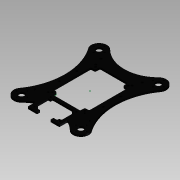
# Autodesk Inventor part: baseatasV2
Saved by Autodesk Inventor 2015 SP1 (Build 190203100, 203)
## iProperties
Created: 2015-01-15
Part Number: baseatasV2
Material: ABS Plastic
Document SubType Name: Modeling
Designer: Rafi Kurnia Putra
Density: 1.06 g/cm^3
Appearance: Smooth - Black
Mass: 28.287 g
Surface Area: 202.895 cm^2
Volume: 26.6858 cm^3
Author: Rafi Kurnia Putra
Autodesk Inventor part; units mm, degrees
ref_plane "YZ Plane" through (0, 0, 0) normal (1, 0, 0) x (0, 1, 0)
ref_plane "XZ Plane" through (0, 0, 0) normal (0, 1, 0) x (-1, 0, 0)
ref_plane "XY Plane" through (0, 0, 0) normal (0, 0, 1) x (1, 0, 0)
sketch "Sketch1" plane through (0, 0, 0) normal (0, 1, 0) x (-1, 0, 0)
  circle A0 centre (-25.375, -42.175) radius 1.75
  circle A1 centre (-25.375, -42.175) radius 1.75
  circle A2 centre (-28.625, -37.55) radius 1.75
  circle A3 centre (-28.625, -37.55) radius 1.75
  circle A4 centre (-25.5, -34.24) radius 1.75
  circle A5 centre (-46.65, -60.8866) radius 4.5
  circle A6 centre (-46.65, -69.3733) radius 1.25
  circle A7 centre (-38.1633, -60.8866) radius 1.25
  circle A8 centre (-55.1367, -60.8866) radius 1.25
  circle A9 centre (-46.65, -52.3999) radius 1.25
  circle A10 centre (-39.5789, -53.8156) radius 1.25
  circle A11 centre (-33.215, -47.4516) radius 1.25
  line L0 (0, -37.55) -> (-19.7877, -37.55)
  line L1 (-21.7877, -35.55) -> (-21.7877, -32)
  line L2 (-28.625, -28) -> (-28.625, 0)
  arc A12 (-28.625, -28) -> (-26.625, -30) centre (-26.625, -28) ccw
  line L3 (-23.7877, -30) -> (-26.625, -30)
  arc A13 (-21.7877, -32) -> (-23.7877, -30) centre (-23.7877, -32) ccw
  arc A14 (-21.7877, -35.55) -> (-19.7877, -37.55) centre (-19.7877, -35.55) ccw
  arc A15 (-21.37, 36.7732) -> (-21.7877, 35.55) centre (-19.7877, 35.55) ccw
  circle A16 centre (-28.625, 37.55) radius 1.75
  circle A17 centre (-28.625, 37.55) radius 1.75
  circle A18 centre (-33.215, 47.4516) radius 1.25
  circle A19 centre (-38.1633, 60.8866) radius 1.25
  circle A20 centre (-39.5789, 53.8156) radius 1.25
  circle A21 centre (-46.65, 52.3999) radius 1.25
  circle A22 centre (-46.65, 69.3733) radius 1.25
  circle A23 centre (-46.65, 60.8866) radius 4.5
  circle A24 centre (-55.1367, 60.8866) radius 1.25
  circle A25 centre (-25.5, 34.24) radius 1.75
  line L4 (-21.7877, 35.55) -> (-21.7877, 32)
  line L5 (-23.7877, 30) -> (-26.625, 30)
  arc A26 (-26.625, 30) -> (-28.625, 28) centre (-26.625, 28) ccw
  line L6 (-28.625, 28) -> (-28.625, 0)
  arc A27 (-23.7877, 30) -> (-21.7877, 32) centre (-23.7877, 32) ccw
  circle A28 centre (-34.6272, 13.8987) radius 1.75
  circle A29 centre (-35.7091, 28.8987) radius 1.75
  circle A30 centre (-25.5, 34.24) radius 1.75
  circle A31 centre (-28.625, 37.55) radius 1.75
  circle A32 centre (-38.6257, 37.55) radius 1.75
  arc A33 (-37.9702, 69.5664) -> (-55.3297, 52.2069) centre (-46.65, 60.8866) ccw
  circle A34 centre (-34.6272, -13.8987) radius 1.75
  circle A35 centre (-25.5, -34.24) radius 1.75
  circle A36 centre (-28.625, -37.55) radius 1.75
  circle A37 centre (-25.375, -42.175) radius 1.75
  arc A38 (-55.3297, -52.2069) -> (-37.9702, -69.5664) centre (-46.65, -60.8866) ccw
  circle A39 centre (-28.8757, 53.55) radius 1.75
  arc A40 (-37.9702, 69.5664) -> (-26.4933, 60.8302) centre (-0.0022, 107.5388) ccw
  arc A41 (0, -40.4412) -> (0, -43.9412) centre (0, -42.1912) ccw
  arc A42 (0, -53.835) -> (-37.9702, -69.5664) centre (0, -107.5245) ccw
  arc A43 (-55.3297, -52.2069) -> (-55.3297, 52.2069) centre (-134.1138, 0) ccw
  arc A44 (0, -46.2631) -> (0, -49.7631) centre (0, -48.0131) ccw
  line L7 (-39.6019, 0) -> (-25.7032, 0) construction
  arc A45 (23.7877, -30) -> (21.7877, -32) centre (23.7877, -32) ccw
  line L8 (28.625, -28) -> (28.625, 0)
  line L9 (21.7877, -35.55) -> (21.7877, -32)
  arc A46 (19.7877, -37.55) -> (21.7877, -35.55) centre (19.7877, -35.55) ccw
  arc A47 (26.625, -30) -> (28.625, -28) centre (26.625, -28) ccw
  circle A48 centre (25.5, -34.24) radius 1.75
  circle A49 centre (28.625, -37.55) radius 1.75
  circle A50 centre (28.625, -37.55) radius 1.75
  circle A51 centre (25.375, -42.175) radius 1.75
  circle A52 centre (25.375, -42.175) radius 1.75
  line L10 (0, -37.55) -> (19.7877, -37.55)
  circle A53 centre (46.65, -60.8866) radius 4.5
  circle A54 centre (46.65, -69.3733) radius 1.25
  circle A55 centre (38.1633, -60.8866) radius 1.25
  circle A56 centre (55.1367, -60.8866) radius 1.25
  circle A57 centre (46.65, -52.3999) radius 1.25
  circle A58 centre (33.215, -47.4516) radius 1.25
  circle A59 centre (39.5789, -53.8156) radius 1.25
  line L11 (23.7877, -30) -> (26.625, -30)
  circle A60 centre (38.1633, 60.8866) radius 1.25
  circle A61 centre (39.5789, 53.8156) radius 1.25
  circle A62 centre (46.65, 52.3999) radius 1.25
  circle A63 centre (55.1367, 60.8866) radius 1.25
  circle A64 centre (46.65, 60.8866) radius 4.5
  circle A65 centre (46.65, 69.3733) radius 1.25
  line L12 (28.625, 28) -> (28.625, 0)
  line L13 (23.7877, 30) -> (26.625, 30)
  arc A66 (28.625, 28) -> (26.625, 30) centre (26.625, 28) ccw
  arc A67 (21.7877, 32) -> (23.7877, 30) centre (23.7877, 32) ccw
  line L14 (21.7877, 35.55) -> (21.7877, 32)
  arc A68 (21.7877, 35.55) -> (21.37, 36.7732) centre (19.7877, 35.55) ccw
  circle A69 centre (25.5, 34.24) radius 1.75
  circle A70 centre (28.625, 37.55) radius 1.75
  circle A71 centre (28.625, 37.55) radius 1.75
  circle A72 centre (33.215, 47.4516) radius 1.25
  arc A73 (55.3297, 52.2069) -> (37.9702, 69.5664) centre (46.65, 60.8866) ccw
  circle A74 centre (25.5, 34.24) radius 1.75
  circle A75 centre (34.6272, 13.8987) radius 1.75
  circle A76 centre (35.7091, 28.8987) radius 1.75
  arc A77 (55.3297, 52.2069) -> (55.3297, -52.2069) centre (134.1138, 0) ccw
  circle A78 centre (34.6272, -13.8987) radius 1.75
  circle A79 centre (28.625, 37.55) radius 1.75
  circle A80 centre (38.6257, 37.55) radius 1.75
  circle A81 centre (25.5, -34.24) radius 1.75
  circle A82 centre (28.625, -37.55) radius 1.75
  circle A83 centre (25.375, -42.175) radius 1.75
  arc A84 (0, -43.9412) -> (0, -40.4412) centre (0, -42.1912) ccw
  arc A85 (37.9702, -69.5664) -> (0, -53.835) centre (0, -107.5245) ccw
  arc A86 (37.9702, -69.5664) -> (55.3297, -52.2069) centre (46.65, -60.8866) ccw
  circle A87 centre (28.8757, 53.55) radius 1.75
  arc A88 (26.4933, 60.8302) -> (37.9702, 69.5664) centre (0.0022, 107.5388) ccw
  arc A89 (0, -49.7631) -> (0, -46.2631) centre (0, -48.0131) ccw
  line L15 (39.6019, 0) -> (25.7032, 0) construction
  line L16 (0, 0) -> (146.4608, 0) construction
  line L17 (-25, 72.1616) -> (-25, 61.7)
  line L18 (-20.5788, 37.1616) -> (20.5788, 37.1616)
  line L19 (25, 61.7) -> (25, 72.1616)
  circle A90 centre (20, 68.1616) radius 1.75
  circle A91 centre (-20, 68.1616) radius 1.75
  circle A92 centre (20, 42.1616) radius 1.75
  circle A93 centre (-20, 42.1616) radius 1.75
  line L20 (10, 72.1616) -> (10, 69.1616)
  line L21 (-10.74, 69.1616) -> (-10.74, 72.1616)
  arc A94 (-26.4933, 60.8302) -> (-25, 61.7) centre (-26, 61.7) ccw
  arc A95 (25, 61.7) -> (26.4933, 60.8302) centre (26, 61.7) ccw
  line L22 (24, 73.1616) -> (11, 73.1616)
  line L23 (-24, 73.1616) -> (-11.74, 73.1616)
  arc A96 (21.37, 36.7732) -> (20.5788, 37.1616) centre (20.5788, 36.1616) ccw
  arc A97 (-20.5788, 37.1616) -> (-21.37, 36.7732) centre (-20.5788, 36.1616) ccw
  line L24 (20, 63.6616) -> (20, 46.6616)
  line L25 (-16.5, 67.1616) -> (-16.5, 65.6616)
  line L26 (-17.5, 64.6616) -> (-19, 64.6616)
  line L27 (-20, 63.6616) -> (-20, 46.6616)
  line L28 (-19, 45.6616) -> (-17.5, 45.6616)
  line L29 (-16.5, 44.6616) -> (-16.5, 43.1616)
  line L30 (-15.5, 42.1616) -> (15.5, 42.1616)
  line L31 (16.5, 43.1616) -> (16.5, 44.6616)
  line L32 (17.5, 45.6616) -> (19, 45.6616)
  line L33 (16.5, 67.1616) -> (16.5, 65.6616)
  line L34 (17.5, 64.6616) -> (19, 64.6616)
  line L35 (15.5, 68.1616) -> (11, 68.1616)
  line L36 (-11.74, 68.1616) -> (-15.5, 68.1616)
  arc A98 (19, 45.6616) -> (20, 46.6616) centre (19, 46.6616) ccw
  arc A99 (17.5, 45.6616) -> (16.5, 44.6616) centre (17.5, 44.6616) ccw
  arc A100 (15.5, 42.1616) -> (16.5, 43.1616) centre (15.5, 43.1616) ccw
  arc A101 (-16.5, 43.1616) -> (-15.5, 42.1616) centre (-15.5, 43.1616) ccw
  arc A102 (-16.5, 44.6616) -> (-17.5, 45.6616) centre (-17.5, 44.6616) ccw
  arc A103 (-20, 46.6616) -> (-19, 45.6616) centre (-19, 46.6616) ccw
  arc A104 (20, 63.6616) -> (19, 64.6616) centre (19, 63.6616) ccw
  arc A105 (16.5, 67.1616) -> (15.5, 68.1616) centre (15.5, 67.1616) ccw
  arc A106 (16.5, 65.6616) -> (17.5, 64.6616) centre (17.5, 65.6616) ccw
  arc A107 (10, 69.1616) -> (11, 68.1616) centre (11, 69.1616) ccw
  arc A108 (11, 73.1616) -> (10, 72.1616) centre (11, 72.1616) ccw
  arc A109 (25, 72.1616) -> (24, 73.1616) centre (24, 72.1616) ccw
  arc A110 (-10.74, 72.1616) -> (-11.74, 73.1616) centre (-11.74, 72.1616) ccw
  arc A111 (-11.74, 68.1616) -> (-10.74, 69.1616) centre (-11.74, 69.1616) ccw
  arc A112 (-15.5, 68.1616) -> (-16.5, 67.1616) centre (-15.5, 67.1616) ccw
  arc A113 (-17.5, 64.6616) -> (-16.5, 65.6616) centre (-17.5, 65.6616) ccw
  arc A114 (-19, 64.6616) -> (-20, 63.6616) centre (-19, 63.6616) ccw
  arc A115 (-24, 73.1616) -> (-25, 72.1616) centre (-24, 72.1616) ccw
  point P0 (-37.9702, -69.5664)
  point P1 (-55.3297, -52.2069)
  point P2 (-4.2075, -54.5249)
  point P3 (-46.65, -60.8866)
  point P4 (-37.9702, 69.5664)
  point P5 (-55.3297, 52.2069)
  point P6 (0.0035, -53.835)
  point P7 (-57.609, 54.4281)
  point P8 (-40.6295, 13.8987)
  point P9 (-40.6295, -13.8987)
  point P10 (55.3297, -52.2069)
  point P11 (37.9702, -69.5664)
  point P12 (37.9702, 69.5664)
  point P13 (55.3297, 52.2069)
  point P14 (46.65, -60.8866)
  point P15 (4.2075, -54.5249)
  point P16 (-0.0035, -53.835)
  point P17 (57.609, 54.4281)
  point P18 (40.6295, 13.8987)
  point P19 (40.6295, -13.8987)
  point P20 (-1.75, -48.0131)
  point P21 (25, 73.1616)
  point P22 (-25, 73.1616)
  point P23 (20.972, 37.1616)
  point P24 (-20.972, 37.1616)
  point P25 (25, 60.0142)
  point P26 (-25, 60.0142)
  point P27 (10, 68.1616)
  point P28 (-10, 68.1616)
  point P29 (10, 73.1616)
  point P30 (-10.74, 73.1616)
  point P31 (10, 68.1616)
  point P32 (20, 45.6616)
  point P33 (20, 64.6616)
  point P34 (16.5, 42.1616)
  point P35 (-16.5, 42.1616)
  point P36 (-16.5, 68.1616)
  point P37 (16.5, 68.1616)
  point P38 (-16.5, 45.6616)
  point P39 (16.5, 45.6616)
  point P40 (46.65, -73.1616)
  point P41 (-58.925, -60.8866)
  point P42 (58.925, -60.8866)
  dimension "d42" = 9
  dimension "d43" = 9
  dimension "d46" = 2.5
  dimension "d86" = 12.0045
  dimension "d87" = 6.0022
  dimension "d88" = 6.0022
  dimension "d92" = 69.2545
  dimension "d93" = 27.7974
  dimension "d94" = 5.8219
  dimension "d95" = 5.8219
  dimension "d97" = 68.48
  dimension "d98" = 51
  dimension "d99" = 9
  dimension "d100" = 8.4867
  dimension "d101" = 2.5
  dimension "d102" = 10
  dimension "d103" = 9
  dimension "d104" = 8.4867
  dimension "d112" = 90
  dimension "d113" = 3.5
  dimension "d114" = 5
  dimension "d116" = 3.5
  dimension "d117" = 5
  dimension "d119" = 3.5
  dimension "d120" = 5
  dimension "d121" = 5
  dimension "d122" = 3.5
  dimension "d123" = 5
  dimension "d124" = 5
  dimension "d126" = 10
  dimension "d133" = 1
  dimension "d137" = 1
  dimension "d138" = 3.5
  dimension "d139" = 3.5
  dimension "d140" = 3.5
  dimension "d141" = 3.5
  dimension "d142" = 1
  dimension "d143" = 3.5
  dimension "d144" = 3.5
  dimension "d145" = 3.5
  dimension "d146" = 1
  dimension "d170" = 146.3233
  dimension "d171" = 117.85
  constraints: 116 centre point, 112 point on circle, 74 end point, 44 tangent, 32 point on line, 18 equal radius, 12 coincident, 11 perpendicular, 6 horizontal, 4 vertical, 4 other
  measures "d42" diameter of A5
  measures "d43" diameter of A23
  measures "d46" diameter of A8
  measures "d86" distance from line of L6 point (-40.629, 13.899)
  measures "d87" distance of A28.centre point (-40.629, 13.899)
  measures "d88" distance of A34.centre point (-40.629, -13.899)
  measures "d92" distance of A28.centre A75.centre
  measures "d93" distance of A78.centre A75.centre
  measures "d94" distance of A44.centre point (0.004, -53.835)
  measures "d95" distance of A84.centre A44.centre
  measures "d97" distance of A81.centre A74.centre
  measures "d98" distance of A25.centre A74.centre
  measures "d99" diameter of A64
  measures "d100" distance of A63.centre A64.centre
  measures "d101" diameter of A63
  measures "d102" distance of A61.centre A64.centre
  measures "d103" distance of A72.centre A61.centre
  measures "d104" distance of A60.centre A73.centre
  measures "d112" angle of L18 L17
  measures "d113" diameter of A90
  measures "d114" distance from line of A90.centre L19
  measures "d116" diameter of A91
  measures "d117" distance from line of L17 A91.centre
  measures "d119" diameter of A92
  measures "d120" distance from line of A92.centre L19
  measures "d121" distance from line of A92.centre L18
  measures "d122" diameter of A93
  measures "d123" distance from line of A93.centre L18
  measures "d124" distance from line of A93.centre L17
  measures "d126" distance of point (-10, 68.162) A91.centre
  measures "d133" radius of A94
  measures "d137" radius of A96
  measures "d138" distance of point (20, 45.662) A92.centre
  measures "d139" distance of point (20, 64.662) A90.centre
  measures "d140" distance of point (16.5, 42.162) A92.centre
  measures "d141" distance of point (-16.5, 42.162) A93.centre
  measures "d142" radius of A98
  measures "d143" distance from line of A91.centre L26
  measures "d144" distance of point (16.5, 68.162) A90.centre
  measures "d145" distance of A91.centre point (-16.5, 68.162)
  measures "d146" radius of A104
  measures "d170" distance from line of point (46.65, -73.162) L22
  measures "d171" distance of point (-58.925, -60.887) point (58.925, -60.887)
extrude "Extrusion6" add sketch "Sketch1" along normal mid plane 3
sketch "Sketch5" plane through (0, 1.5, 0) normal (0, 1, 0) x (1, 0, 0)
  line L0 (-68.183, -17.0535) -> (-47.8943, -30.2678)
  arc A0 (-46.3635, -35.1053) -> (-46.3635, 35.1053) centre (-134.1138, 0) ccw
  line L1 (-68.183, 17.0535) -> (-47.8943, 30.2678)
  arc A1 (-46.3635, -35.1053) -> (-47.8943, -30.2678) centre (-50.0774, -33.6196) ccw
  arc A2 (-47.8943, 30.2678) -> (-46.3635, 35.1053) centre (-50.0774, 33.6196) ccw
  line L2 (0, -8.7241) -> (0, 8.1787)
  line L3 (-70, -13.7017) -> (-70, 13.7017)
  arc A3 (-68.183, 17.0535) -> (-70, 13.7017) centre (-66, 13.7017) ccw
  arc A4 (-70, -13.7017) -> (-68.183, -17.0535) centre (-66, -13.7017) ccw
  line L4 (68.183, -17.0535) -> (47.8943, -30.2678)
  arc A5 (46.3635, 35.1053) -> (46.3635, -35.1053) centre (134.1138, 0) ccw
  line L5 (68.183, 17.0535) -> (47.8943, 30.2678)
  arc A6 (47.8943, -30.2678) -> (46.3635, -35.1053) centre (50.0774, -33.6196) ccw
  arc A7 (46.3635, 35.1053) -> (47.8943, 30.2678) centre (50.0774, 33.6196) ccw
  line L6 (70, -13.7017) -> (70, 13.7017)
  arc A8 (70, 13.7017) -> (68.183, 17.0535) centre (66, 13.7017) ccw
  arc A9 (68.183, -17.0535) -> (70, -13.7017) centre (66, -13.7017) ccw
  point P0 (0, 0)
  point P1 (-45.1937, -32.0268)
  point P2 (-70, 0)
  point P3 (45.1937, -32.0268)
  point P4 (70, 0)
  dimension "d150" = 4
  dimension "d154" = 70
  dimension "d155" = 4
  constraints: 20 point on circle, 15 symmetric about line, 14 end point, 10 centre point, 6 tangent, 3 vertical, 2 equal radius, 2 point on line, 5 other
  measures "d150" radius of A1
  measures "d154" distance from line of point (-70, 0) L2
  measures "d155" radius of A3
sketch "Sketch7" plane through (0, 1.5, 0) normal (0, 1, 0) x (1, 0, 0)
  arc A0 (0, 53.835) -> (37.9702, 69.5664) centre (0, 107.5245) ccw
  arc A1 (-37.9702, 69.5664) -> (0, 53.835) centre (0, 107.5245) ccw
  arc A2 (46.65, 73.1616) -> (37.9702, 69.5664) centre (46.65, 60.8866) ccw
  arc A3 (-37.9702, 69.5664) -> (-46.65, 73.1616) centre (-46.65, 60.8866) ccw
  line L0 (46.65, 73.1616) -> (-46.65, 73.1616)
  constraints: 8 point on circle, 4 centre point, 2 end point, 1 horizontal
sketch "Sketch8" plane through (0, 1.5, 0) normal (0, 1, 0) x (1, 0, 0)
  arc A0 (55.3297, 52.2069) -> (55.3297, -52.2069) centre (134.1138, 0) ccw projected
  circle A1 centre (55.1367, -60.8866) radius 1.25 projected
  circle A2 centre (-55.1367, -60.8866) radius 1.25 projected
  arc A3 (-55.3297, -52.2069) -> (-37.9702, -69.5664) centre (-46.65, -60.8866) ccw projected
  circle A4 centre (46.65, 69.3733) radius 1.25 projected
  arc A5 (55.3297, 52.2069) -> (37.9702, 69.5664) centre (46.65, 60.8866) ccw projected
  line L0 (11.74, -73.1616) -> (24, -73.1616) projected
  circle A6 centre (35.7091, -28.8987) radius 1.75 projected
  circle A7 centre (-35.7091, -28.8987) radius 1.75 projected
  line L1 (0, 0) -> (-2.9258, 0)
  circle A8 centre (35.7091, 28.8987) radius 1.75
  circle A9 centre (-35.7091, 28.8987) radius 1.75
  circle A10 centre (38.6257, -37.55) radius 1.75 projected
  circle A11 centre (-38.6257, -37.55) radius 1.75 projected
  circle A12 centre (38.6257, 37.55) radius 1.75
  circle A13 centre (-38.6257, 37.55) radius 1.75
  point P0 (39.6019, 0)
  point P1 (-39.6104, 0)
  point P2 (58.8841, -60.8866)
  point P3 (-58.925, -60.8866)
  point P4 (46.694, 73.1615)
  dimension "d163" = 79.2123
  dimension "d164" = 117.809
  dimension "d165" = 146.3232
  constraints: 4 centre point, 4 symmetric about line, 3 point on circle, 2 end point, 1 horizontal, 4 other
  measures "d163" distance of point (-39.61, 0) point (39.602, 0)
  measures "d164" distance of point (58.884, -60.887) point (-58.925, -60.887)
  measures "d165" distance from line of L0 point (46.694, 73.162)
extrude "Extrusion11" cut sketch "Sketch8" against normal through all contours A8 | A9 | A12 | A13
sketch "Sketch10" plane through (0, 1.5, 0) normal (0, 1, 0) x (1, 0, 0)
  circle A0 centre (35.7091, -28.8987) radius 1.75 projected
  circle A1 centre (38.6257, -37.55) radius 1.75 projected
  circle A2 centre (-38.6257, -37.55) radius 1.75 projected
  circle A3 centre (-35.7091, -28.8987) radius 1.75 projected
  circle A4 centre (-35.7091, 28.8987) radius 1.75 projected
  circle A5 centre (-38.6257, 37.55) radius 1.75 projected
  circle A6 centre (35.7091, 28.8987) radius 1.75 projected
  circle A7 centre (38.6257, 37.55) radius 1.75 projected
  point P0 (0, 0)
extrude "Extrusion12" add sketch "Sketch10" against normal blind 3
sketch "Sketch12" plane through (0, 1.5, 0) normal (0, 1, 0) x (1, 0, 0)
  arc A0 (-37.9702, 69.5664) -> (-55.3297, 52.2069) centre (-46.65, 60.8866) ccw projected
  line L0 (-24, -73.1616) -> (-11, -73.1616) projected
  arc A1 (-55.3297, -52.2069) -> (-37.9702, -69.5664) centre (-46.65, -60.8866) ccw projected
  arc A2 (37.9702, -69.5664) -> (55.3297, -52.2069) centre (46.65, -60.8866) ccw projected
  circle A3 centre (-37.5, -40) radius 1.75
  circle A4 centre (-28.625, -37.55) radius 1.75 projected
  line L1 (0, 0) -> (0, 1.0558)
  line L2 (0, 0) -> (1.0558, 0) construction
  circle A5 centre (-37.5, 40) radius 1.75
  line L3 (0, 0) -> (0, -1.0558)
  circle A6 centre (37.5, -40) radius 1.75
  circle A7 centre (37.5, 40) radius 1.75
  point P0 (-46.65, 73.1616)
  point P1 (-58.925, -60.8866)
  point P2 (58.925, -60.8866)
  dimension "d181" = 146.3233
  dimension "d182" = 117.85
  dimension "d183" = 3.5
  dimension "d186" = 40
  dimension "d187" = 37.5
  dimension "d190" = 90
  constraints: 6 end point, 4 centre point, 4 symmetric about line, 3 point on circle, 1 horizontal, 1 perpendicular, 3 other
  measures "d181" distance from line of L0 point (-46.65, 73.162)
  measures "d182" distance of point (-58.925, -60.887) point (58.925, -60.887)
  measures "d183" diameter of A3
  measures "d186" vertical distance of L1.start A3.centre
  measures "d187" horizontal distance of A3.centre L1.start
  measures "d190" angle of L2 L1
sketch "Sketch14" plane through (0, 1.5, 0) normal (0, 1, 0) x (1, 0, 0)
  circle A0 centre (-43, -44.1209) radius 1.75
  circle A1 centre (43, -44.1209) radius 1.75
  circle A2 centre (-34.28, 40.8791) radius 1.75
  circle A3 centre (34.28, 40.8791) radius 1.75
  arc A4 (-55.3297, -52.2069) -> (-37.9702, -69.5664) centre (-46.65, -60.8866) ccw projected
  circle A5 centre (-46.65, -60.8866) radius 4.5 projected
  circle A6 centre (-46.65, -60.8866) radius 12.275
  arc A7 (37.9702, -69.5664) -> (55.3297, -52.2069) centre (46.65, -60.8866) ccw projected
  circle A8 centre (46.65, -60.8866) radius 4.5 projected
  circle A9 centre (46.65, -60.8866) radius 12.275
  point P0 (0, 0)
  point P1 (0, 0)
  dimension "d198" = 43
  dimension "d199" = 85
  dimension "d200" = 43
  dimension "d201" = 85
  constraints: 6 centre point, 2 coincident, 2 other
  measures "d198" horizontal distance of A1.centre point (0, 0)
  measures "d199" vertical distance of A3.centre A1.centre
  measures "d200" horizontal distance of A0.centre point (0, 0)
  measures "d201" vertical distance of A2.centre A0.centre
extrude "Extrusion16" cut sketch "Sketch14" against normal through all contours A0 | A1 | A2 | A3
sketch "Sketch15" plane through (0, 1.5, 0) normal (0, 1, 0) x (1, 0, 0)
  circle A0 centre (-23.8036, 38.7811) radius 1.75 projected
  circle A1 centre (-87.5709, 50.7669) radius 1.75 projected
  point P0 (0, 0)
extrude "Extrusion17" cut sketch "Sketch15" against normal up to next
sketch "Sketch16" plane through (0, 1.5, 0) normal (0, 1, 0) x (1, 0, 0)
  circle A0 centre (-39.5789, -53.8156) radius 1.25 projected
  circle A1 centre (-33.215, -47.4516) radius 1.25 projected
  circle A2 centre (33.215, -47.4516) radius 1.25 projected
  circle A3 centre (39.5789, -53.8156) radius 1.25 projected
  arc A4 (32.1247, 48.063) -> (33.7243, 48.5931) centre (33.215, 47.4516) ccw
  circle A5 centre (39.5789, 53.8156) radius 1.25 projected
  arc A6 (-33.7243, 48.5931) -> (-32.1247, 48.063) centre (-33.215, 47.4516) ccw
  arc A7 (-33.7243, 48.5931) -> (-32.1247, 48.063) centre (-32.442, 49.784) ccw
  arc A8 (32.1247, 48.063) -> (33.7243, 48.5931) centre (32.442, 49.784) ccw
  circle A9 centre (-39.5789, 53.8156) radius 1.25 projected
  circle A10 centre (32.442, 49.784) radius 1.75
  circle A11 centre (-32.442, 49.784) radius 1.75
  point P0 (0, 0)
  constraints: 8 point on circle, 6 centre point, 2 coincident
extrude "Extrusion18" add sketch "Sketch16" against normal blind 3 contours A0 | A1 | A2 | A3 | A8 A4 | A5 | A7 A6 | A9
extrude "Extrusion19" cut sketch "Sketch16" against normal up to next contours A10 A8 | A11 A7
sketch "Sketch18" plane through (0, 1.5, 0) normal (0, 1, 0) x (1, 0, 0)
  circle A0 centre (34.6272, -13.8987) radius 1.75 projected
  circle A1 centre (43, -44.1209) radius 1.75 projected
  circle A2 centre (34.6272, 13.8987) radius 1.75 projected
  circle A3 centre (34.28, 40.8791) radius 1.75 projected
  circle A4 centre (-34.28, 40.8791) radius 1.75 projected
  circle A5 centre (-34.6272, 13.8987) radius 1.75 projected
  circle A6 centre (-34.6272, -13.8987) radius 1.75 projected
  circle A7 centre (-43, -44.1209) radius 1.75 projected
  point P0 (0, 0)
  dimension "d208" = 30.2221
  dimension "d209" = 8.3728
  dimension "d210" = 26.9804
  dimension "d211" = 0.3472
  measures "d208" vertical distance of A6.centre A7.centre
  measures "d209" horizontal distance of A6.centre A7.centre
  measures "d210" vertical distance of A4.centre A5.centre
  measures "d211" horizontal distance of A4.centre A5.centre
sketch "Sketch19" plane through (0, 1.5, 0) normal (0, 1, 0) x (1, 0, 0)
  circle A0 centre (-28.8757, -53.55) radius 1.75 projected
  circle A1 centre (28.8757, -53.55) radius 1.75 projected
  circle A2 centre (34.28, 40.8791) radius 1.75 projected
  circle A3 centre (25.375, 42.175) radius 1.75 projected
  circle A4 centre (-23.8036, 38.7811) radius 1.75 projected
  circle A5 centre (-25.375, 42.175) radius 1.75 projected
  circle A6 centre (-34.28, 40.8791) radius 1.75 projected
  arc A7 (0, 40.4412) -> (0, 43.9412) centre (0, 42.1912) ccw projected
  arc A8 (0, 43.9412) -> (0, 40.4412) centre (0, 42.1912) ccw projected
  circle A9 centre (0, 48.0131) radius 1.75 projected
  point P0 (0, 0)
extrude "Extrusion20" add sketch "Sketch19" against normal blind 3
sketch "Sketch20" plane through (0, 1.5, 0) normal (0, 1, 0) x (1, 0, 0)
  circle A0 centre (-43, -44.1209) radius 1.75 projected
  circle A1 centre (43, -44.1209) radius 1.75 projected
  arc A2 (21.7877, 35.55) -> (19.7877, 37.55) centre (19.7877, 35.55) ccw projected
  line L0 (21.7877, 35.55) -> (21.7877, 32) projected
  arc A3 (21.7877, 32) -> (23.7877, 30) centre (23.7877, 32) ccw projected
  line L1 (23.7877, 30) -> (26.625, 30) projected
  arc A4 (28.625, 28) -> (26.625, 30) centre (26.625, 28) ccw projected
  line L2 (28.625, 28) -> (28.625, -28) projected
  arc A5 (26.625, -30) -> (28.625, -28) centre (26.625, -28) ccw projected
  line L3 (26.625, -30) -> (23.7877, -30) projected
  arc A6 (23.7877, -30) -> (21.7877, -32) centre (23.7877, -32) ccw projected
  line L4 (21.7877, -32) -> (21.7877, -35.55) projected
  arc A7 (21.37, -36.7732) -> (21.7877, -35.55) centre (19.7877, -35.55) ccw projected
  arc A8 (20.5788, -37.1616) -> (21.37, -36.7732) centre (20.5788, -36.1616) ccw projected
  line L5 (20.5788, -37.1616) -> (-20.5788, -37.1616) projected
  arc A9 (-21.37, -36.7732) -> (-20.5788, -37.1616) centre (-20.5788, -36.1616) ccw projected
  arc A10 (-21.7877, -35.55) -> (-21.37, -36.7732) centre (-19.7877, -35.55) ccw projected
  line L6 (-21.7877, -35.55) -> (-21.7877, -32) projected
  arc A11 (-21.7877, -32) -> (-23.7877, -30) centre (-23.7877, -32) ccw projected
  line L7 (-23.7877, -30) -> (-26.625, -30) projected
  arc A12 (-28.625, -28) -> (-26.625, -30) centre (-26.625, -28) ccw projected
  line L8 (-28.625, -28) -> (-28.625, 28) projected
  arc A13 (-26.625, 30) -> (-28.625, 28) centre (-26.625, 28) ccw projected
  line L9 (-26.625, 30) -> (-23.7877, 30) projected
  arc A14 (-23.7877, 30) -> (-21.7877, 32) centre (-23.7877, 32) ccw projected
  line L10 (-21.7877, 32) -> (-21.7877, 35.55) projected
  arc A15 (-19.7877, 37.55) -> (-21.7877, 35.55) centre (-19.7877, 35.55) ccw projected
  line L11 (-19.7877, 37.55) -> (19.7877, 37.55) projected
  circle A16 centre (-46.65, 60.8866) radius 4.5 projected
  circle A17 centre (-46.65, -60.8866) radius 4.5 projected
  circle A18 centre (46.65, -60.8866) radius 4.5 projected
  circle A19 centre (46.65, 60.8866) radius 4.5 projected
  circle A20 centre (20, -42.1616) radius 1.75 projected
  circle A21 centre (-20, -42.1616) radius 1.75 projected
  circle A22 centre (20, -68.1616) radius 1.75 projected
  circle A23 centre (-20, -68.1616) radius 1.75 projected
  circle A24 centre (-34.6272, 13.8987) radius 1.75 projected
  circle A25 centre (-25.5, 34.24) radius 1.75 projected
  circle A26 centre (-28.625, 37.55) radius 1.75 projected
  circle A27 centre (-28.625, -37.55) radius 1.75 projected
  circle A28 centre (-25.5, -34.24) radius 1.75 projected
  circle A29 centre (-34.6272, -13.8987) radius 1.75 projected
  circle A30 centre (34.6272, 13.8987) radius 1.75 projected
  circle A31 centre (34.6272, -13.8987) radius 1.75 projected
  circle A32 centre (25.5, -34.24) radius 1.75 projected
  circle A33 centre (28.625, -37.55) radius 1.75 projected
  circle A34 centre (25.5, 34.24) radius 1.75 projected
  circle A35 centre (28.625, 37.55) radius 1.75 projected
  circle A36 centre (-55.1367, 60.8866) radius 1.25 projected
  circle A37 centre (-38.1633, 60.8866) radius 1.25 projected
  circle A38 centre (-46.65, 69.3733) radius 1.25 projected
  circle A39 centre (-46.65, -69.3733) radius 1.25 projected
  circle A40 centre (-55.1367, -60.8866) radius 1.25 projected
  circle A41 centre (-38.1633, -60.8866) radius 1.25 projected
  circle A42 centre (-46.65, 52.3999) radius 1.25 projected
  circle A43 centre (-32.442, 49.784) radius 1.75 projected
  circle A44 centre (-46.65, -52.3999) radius 1.25 projected
  circle A45 centre (46.65, -69.3733) radius 1.25 projected
  circle A46 centre (55.1367, -60.8866) radius 1.25 projected
  circle A47 centre (46.65, -52.3999) radius 1.25 projected
  circle A48 centre (38.1633, -60.8866) radius 1.25 projected
  circle A49 centre (32.442, 49.784) radius 1.75 projected
  circle A50 centre (46.65, 52.3999) radius 1.25 projected
  circle A51 centre (55.1367, 60.8866) radius 1.25 projected
  circle A52 centre (38.1633, 60.8866) radius 1.25 projected
  circle A53 centre (46.65, 69.3733) radius 1.25 projected
  arc A54 (37.9702, -69.5664) -> (55.3297, -52.2069) centre (46.65, -60.8866) ccw projected
  arc A55 (55.3297, 52.2069) -> (55.3297, -52.2069) centre (134.1138, 0) ccw projected
  arc A56 (55.3297, 52.2069) -> (37.9702, 69.5664) centre (46.65, 60.8866) ccw projected
  arc A57 (0, 53.835) -> (37.9702, 69.5664) centre (0, 107.5245) ccw projected
  arc A58 (-37.9702, 69.5664) -> (0, 53.835) centre (0, 107.5245) ccw projected
  arc A59 (-37.9702, 69.5664) -> (-55.3297, 52.2069) centre (-46.65, 60.8866) ccw projected
  arc A60 (-55.3297, -52.2069) -> (-55.3297, 52.2069) centre (-134.1138, 0) ccw projected
  arc A61 (-55.3297, -52.2069) -> (-37.9702, -69.5664) centre (-46.65, -60.8866) ccw projected
  arc A62 (-26.4933, -60.8302) -> (-37.9702, -69.5664) centre (-0.0022, -107.5388) ccw projected
  arc A63 (-25, -61.7) -> (-26.4933, -60.8302) centre (-26, -61.7) ccw projected
  line L12 (-25, -61.7) -> (-25, -72.1616) projected
  arc A64 (-25, -72.1616) -> (-24, -73.1616) centre (-24, -72.1616) ccw projected
  line L13 (-24, -73.1616) -> (-11, -73.1616) projected
  arc A65 (-11, -73.1616) -> (-10, -72.1616) centre (-11, -72.1616) ccw projected
  line L14 (-10, -72.1616) -> (-10, -69.1616) projected
  arc A66 (-10, -69.1616) -> (-11, -68.1616) centre (-11, -69.1616) ccw projected
  line L15 (-11, -68.1616) -> (-15.5, -68.1616) projected
  arc A67 (-16.5, -67.1616) -> (-15.5, -68.1616) centre (-15.5, -67.1616) ccw projected
  line L16 (-16.5, -67.1616) -> (-16.5, -65.6616) projected
  arc A68 (-16.5, -65.6616) -> (-17.5, -64.6616) centre (-17.5, -65.6616) ccw projected
  line L17 (-17.5, -64.6616) -> (-19, -64.6616) projected
  arc A69 (-20, -63.6616) -> (-19, -64.6616) centre (-19, -63.6616) ccw projected
  line L18 (-20, -63.6616) -> (-20, -46.6616) projected
  arc A70 (-19, -45.6616) -> (-20, -46.6616) centre (-19, -46.6616) ccw projected
  line L19 (-19, -45.6616) -> (-17.5, -45.6616) projected
  arc A71 (-17.5, -45.6616) -> (-16.5, -44.6616) centre (-17.5, -44.6616) ccw projected
  line L20 (-16.5, -44.6616) -> (-16.5, -43.1616) projected
  arc A72 (-15.5, -42.1616) -> (-16.5, -43.1616) centre (-15.5, -43.1616) ccw projected
  line L21 (-15.5, -42.1616) -> (15.5, -42.1616) projected
  arc A73 (16.5, -43.1616) -> (15.5, -42.1616) centre (15.5, -43.1616) ccw projected
  line L22 (16.5, -43.1616) -> (16.5, -44.6616) projected
  arc A74 (16.5, -44.6616) -> (17.5, -45.6616) centre (17.5, -44.6616) ccw projected
  line L23 (17.5, -45.6616) -> (19, -45.6616) projected
  arc A75 (20, -46.6616) -> (19, -45.6616) centre (19, -46.6616) ccw projected
  line L24 (20, -46.6616) -> (20, -63.6616) projected
  arc A76 (19, -64.6616) -> (20, -63.6616) centre (19, -63.6616) ccw projected
  line L25 (19, -64.6616) -> (17.5, -64.6616) projected
  arc A77 (17.5, -64.6616) -> (16.5, -65.6616) centre (17.5, -65.6616) ccw projected
  line L26 (16.5, -65.6616) -> (16.5, -67.1616) projected
  arc A78 (15.5, -68.1616) -> (16.5, -67.1616) centre (15.5, -67.1616) ccw projected
  line L27 (15.5, -68.1616) -> (11.74, -68.1616) projected
  arc A79 (11.74, -68.1616) -> (10.74, -69.1616) centre (11.74, -69.1616) ccw projected
  line L28 (10.74, -69.1616) -> (10.74, -72.1616) projected
  arc A80 (10.74, -72.1616) -> (11.74, -73.1616) centre (11.74, -72.1616) ccw projected
  line L29 (11.74, -73.1616) -> (24, -73.1616) projected
  arc A81 (24, -73.1616) -> (25, -72.1616) centre (24, -72.1616) ccw projected
  line L30 (25, -72.1616) -> (25, -61.7) projected
  arc A82 (26.4933, -60.8302) -> (25, -61.7) centre (26, -61.7) ccw projected
  arc A83 (37.9702, -69.5664) -> (26.4933, -60.8302) centre (0.0022, -107.5388) ccw projected
  point P0 (0, 0)
sketch "Sketch21" plane through (0, 1.5, 0) normal (0, 1, 0) x (1, 0, 0)
  circle A0 centre (-43, -44.1209) radius 1.75 projected
  circle A1 centre (43, -44.1209) radius 1.75 projected
  arc A2 (21.7877, 35.55) -> (19.7877, 37.55) centre (19.7877, 35.55) ccw projected
  line L0 (21.7877, 35.55) -> (21.7877, 32) projected
  arc A3 (21.7877, 32) -> (23.7877, 30) centre (23.7877, 32) ccw projected
  line L1 (23.7877, 30) -> (26.625, 30) projected
  arc A4 (28.625, 28) -> (26.625, 30) centre (26.625, 28) ccw projected
  line L2 (28.625, 28) -> (28.625, -28) projected
  arc A5 (26.625, -30) -> (28.625, -28) centre (26.625, -28) ccw projected
  line L3 (26.625, -30) -> (23.7877, -30) projected
  arc A6 (23.7877, -30) -> (21.7877, -32) centre (23.7877, -32) ccw projected
  line L4 (21.7877, -32) -> (21.7877, -35.55) projected
  arc A7 (21.37, -36.7732) -> (21.7877, -35.55) centre (19.7877, -35.55) ccw projected
  arc A8 (20.5788, -37.1616) -> (21.37, -36.7732) centre (20.5788, -36.1616) ccw projected
  line L5 (20.5788, -37.1616) -> (-20.5788, -37.1616) projected
  arc A9 (-21.37, -36.7732) -> (-20.5788, -37.1616) centre (-20.5788, -36.1616) ccw projected
  arc A10 (-21.7877, -35.55) -> (-21.37, -36.7732) centre (-19.7877, -35.55) ccw projected
  line L6 (-21.7877, -35.55) -> (-21.7877, -32) projected
  arc A11 (-21.7877, -32) -> (-23.7877, -30) centre (-23.7877, -32) ccw projected
  line L7 (-23.7877, -30) -> (-26.625, -30) projected
  arc A12 (-28.625, -28) -> (-26.625, -30) centre (-26.625, -28) ccw projected
  line L8 (-28.625, -28) -> (-28.625, 28) projected
  arc A13 (-26.625, 30) -> (-28.625, 28) centre (-26.625, 28) ccw projected
  line L9 (-26.625, 30) -> (-23.7877, 30) projected
  arc A14 (-23.7877, 30) -> (-21.7877, 32) centre (-23.7877, 32) ccw projected
  line L10 (-21.7877, 32) -> (-21.7877, 35.55) projected
  arc A15 (-19.7877, 37.55) -> (-21.7877, 35.55) centre (-19.7877, 35.55) ccw projected
  line L11 (-19.7877, 37.55) -> (19.7877, 37.55) projected
  circle A16 centre (-46.65, 60.8866) radius 4.5 projected
  circle A17 centre (-46.65, -60.8866) radius 4.5 projected
  circle A18 centre (46.65, -60.8866) radius 4.5 projected
  circle A19 centre (46.65, 60.8866) radius 4.5 projected
  circle A20 centre (20, -42.1616) radius 1.75 projected
  circle A21 centre (-20, -42.1616) radius 1.75 projected
  circle A22 centre (20, -68.1616) radius 1.75 projected
  circle A23 centre (-20, -68.1616) radius 1.75 projected
  circle A24 centre (-34.6272, 13.8987) radius 1.75 projected
  circle A25 centre (-25.5, 34.24) radius 1.75 projected
  circle A26 centre (-28.625, 37.55) radius 1.75 projected
  circle A27 centre (-28.625, -37.55) radius 1.75 projected
  circle A28 centre (-25.5, -34.24) radius 1.75 projected
  circle A29 centre (-34.6272, -13.8987) radius 1.75 projected
  circle A30 centre (34.6272, 13.8987) radius 1.75 projected
  circle A31 centre (34.6272, -13.8987) radius 1.75 projected
  circle A32 centre (25.5, -34.24) radius 1.75 projected
  circle A33 centre (28.625, -37.55) radius 1.75 projected
  circle A34 centre (25.5, 34.24) radius 1.75 projected
  circle A35 centre (28.625, 37.55) radius 1.75 projected
  circle A36 centre (-55.1367, 60.8866) radius 1.25 projected
  circle A37 centre (-38.1633, 60.8866) radius 1.25 projected
  circle A38 centre (-46.65, 69.3733) radius 1.25 projected
  circle A39 centre (-46.65, -69.3733) radius 1.25 projected
  circle A40 centre (-55.1367, -60.8866) radius 1.25 projected
  circle A41 centre (-38.1633, -60.8866) radius 1.25 projected
  circle A42 centre (-46.65, 52.3999) radius 1.25 projected
  circle A43 centre (-32.442, 49.784) radius 1.75 projected
  circle A44 centre (-46.65, -52.3999) radius 1.25 projected
  circle A45 centre (46.65, -69.3733) radius 1.25 projected
  circle A46 centre (55.1367, -60.8866) radius 1.25 projected
  circle A47 centre (46.65, -52.3999) radius 1.25 projected
  circle A48 centre (38.1633, -60.8866) radius 1.25 projected
  circle A49 centre (32.442, 49.784) radius 1.75 projected
  circle A50 centre (46.65, 52.3999) radius 1.25 projected
  circle A51 centre (55.1367, 60.8866) radius 1.25 projected
  circle A52 centre (38.1633, 60.8866) radius 1.25 projected
  circle A53 centre (46.65, 69.3733) radius 1.25 projected
  arc A54 (37.9702, -69.5664) -> (55.3297, -52.2069) centre (46.65, -60.8866) ccw projected
  arc A55 (55.3297, 52.2069) -> (55.3297, -52.2069) centre (134.1138, 0) ccw projected
  arc A56 (55.3297, 52.2069) -> (37.9702, 69.5664) centre (46.65, 60.8866) ccw projected
  arc A57 (0, 53.835) -> (37.9702, 69.5664) centre (0, 107.5245) ccw projected
  arc A58 (-37.9702, 69.5664) -> (0, 53.835) centre (0, 107.5245) ccw projected
  arc A59 (-37.9702, 69.5664) -> (-55.3297, 52.2069) centre (-46.65, 60.8866) ccw projected
  arc A60 (-55.3297, -52.2069) -> (-55.3297, 52.2069) centre (-134.1138, 0) ccw projected
  arc A61 (-55.3297, -52.2069) -> (-37.9702, -69.5664) centre (-46.65, -60.8866) ccw projected
  arc A62 (-26.4933, -60.8302) -> (-37.9702, -69.5664) centre (-0.0022, -107.5388) ccw projected
  arc A63 (-25, -61.7) -> (-26.4933, -60.8302) centre (-26, -61.7) ccw projected
  line L12 (-25, -61.7) -> (-25, -72.1616) projected
  arc A64 (-25, -72.1616) -> (-24, -73.1616) centre (-24, -72.1616) ccw projected
  line L13 (-24, -73.1616) -> (-11, -73.1616) projected
  arc A65 (-11, -73.1616) -> (-10, -72.1616) centre (-11, -72.1616) ccw projected
  line L14 (-10, -72.1616) -> (-10, -69.1616) projected
  arc A66 (-10, -69.1616) -> (-11, -68.1616) centre (-11, -69.1616) ccw projected
  line L15 (-11, -68.1616) -> (-15.5, -68.1616) projected
  arc A67 (-16.5, -67.1616) -> (-15.5, -68.1616) centre (-15.5, -67.1616) ccw projected
  line L16 (-16.5, -67.1616) -> (-16.5, -65.6616) projected
  arc A68 (-16.5, -65.6616) -> (-17.5, -64.6616) centre (-17.5, -65.6616) ccw projected
  line L17 (-17.5, -64.6616) -> (-19, -64.6616) projected
  arc A69 (-20, -63.6616) -> (-19, -64.6616) centre (-19, -63.6616) ccw projected
  line L18 (-20, -63.6616) -> (-20, -46.6616) projected
  arc A70 (-19, -45.6616) -> (-20, -46.6616) centre (-19, -46.6616) ccw projected
  line L19 (-19, -45.6616) -> (-17.5, -45.6616) projected
  arc A71 (-17.5, -45.6616) -> (-16.5, -44.6616) centre (-17.5, -44.6616) ccw projected
  line L20 (-16.5, -44.6616) -> (-16.5, -43.1616) projected
  arc A72 (-15.5, -42.1616) -> (-16.5, -43.1616) centre (-15.5, -43.1616) ccw projected
  line L21 (-15.5, -42.1616) -> (15.5, -42.1616) projected
  arc A73 (16.5, -43.1616) -> (15.5, -42.1616) centre (15.5, -43.1616) ccw projected
  line L22 (16.5, -43.1616) -> (16.5, -44.6616) projected
  arc A74 (16.5, -44.6616) -> (17.5, -45.6616) centre (17.5, -44.6616) ccw projected
  line L23 (17.5, -45.6616) -> (19, -45.6616) projected
  arc A75 (20, -46.6616) -> (19, -45.6616) centre (19, -46.6616) ccw projected
  line L24 (20, -46.6616) -> (20, -63.6616) projected
  arc A76 (19, -64.6616) -> (20, -63.6616) centre (19, -63.6616) ccw projected
  line L25 (19, -64.6616) -> (17.5, -64.6616) projected
  arc A77 (17.5, -64.6616) -> (16.5, -65.6616) centre (17.5, -65.6616) ccw projected
  line L26 (16.5, -65.6616) -> (16.5, -67.1616) projected
  arc A78 (15.5, -68.1616) -> (16.5, -67.1616) centre (15.5, -67.1616) ccw projected
  line L27 (15.5, -68.1616) -> (11.74, -68.1616) projected
  arc A79 (11.74, -68.1616) -> (10.74, -69.1616) centre (11.74, -69.1616) ccw projected
  line L28 (10.74, -69.1616) -> (10.74, -72.1616) projected
  arc A80 (10.74, -72.1616) -> (11.74, -73.1616) centre (11.74, -72.1616) ccw projected
  line L29 (11.74, -73.1616) -> (24, -73.1616) projected
  arc A81 (24, -73.1616) -> (25, -72.1616) centre (24, -72.1616) ccw projected
  line L30 (25, -72.1616) -> (25, -61.7) projected
  arc A82 (26.4933, -60.8302) -> (25, -61.7) centre (26, -61.7) ccw projected
  arc A83 (37.9702, -69.5664) -> (26.4933, -60.8302) centre (0.0022, -107.5388) ccw projected
  point P0 (0, 0)
sketch "Sketch22" plane through (0, -1.5, 0) normal (0, -1, 0) x (1, 0, 0)
  circle A0 centre (25.5, 34.24) radius 1.75 projected
  circle A1 centre (-25.5, 34.24) radius 1.75 projected
  line L0 (-20.5788, 37.1616) -> (20.5788, 37.1616) projected
  line L1 (23.7877, 30) -> (26.625, 30) projected
  arc A2 (21.7877, 32) -> (23.7877, 30) centre (23.7877, 32) ccw projected
  line L2 (21.7877, 35.55) -> (21.7877, 32) projected
  arc A3 (21.7877, 35.55) -> (21.37, 36.7732) centre (19.7877, 35.55) ccw projected
  arc A4 (21.37, 36.7732) -> (20.5788, 37.1616) centre (20.5788, 36.1616) ccw projected
  arc A5 (28.625, 28) -> (26.625, 30) centre (26.625, 28) ccw projected
  line L3 (-21.7877, 32) -> (-21.7877, 35.55) projected
  arc A6 (-21.37, 36.7732) -> (-21.7877, 35.55) centre (-19.7877, 35.55) ccw projected
  arc A7 (-20.5788, 37.1616) -> (-21.37, 36.7732) centre (-20.5788, 36.1616) ccw projected
  arc A8 (-23.7877, 30) -> (-21.7877, 32) centre (-23.7877, 32) ccw projected
  line L4 (-26.625, 30) -> (-23.7877, 30) projected
  arc A9 (-26.625, 30) -> (-28.625, 28) centre (-26.625, 28) ccw projected
  point P0 (0, 0)
body "Solid4"
